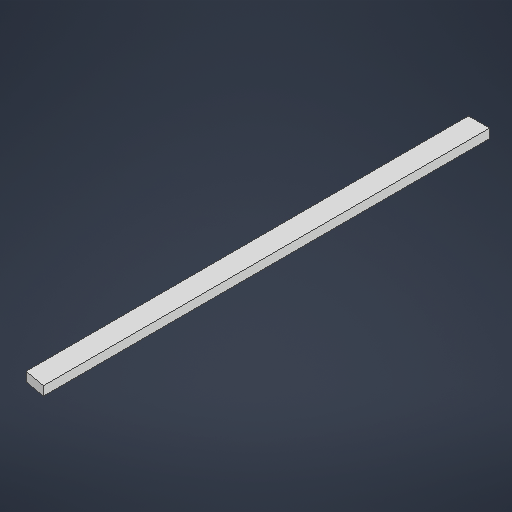
# Autodesk Inventor part: S_2x4x82
Saved by Autodesk Inventor 2027.1 (Build 311270010, 270A)
## iProperties
Created: 2026-09-01
Part Number: S_2x4x82
Material: Generic
Document SubType Name: Modeling
Designer: jorda
Density: 1 g/cm^3
Appearance: Default
Author: jorda
Autodesk Inventor part; units mm, degrees
ref_plane "YZ Plane" through (0, 0, 0) normal (1, 0, 0) x (0, 1, 0)
ref_plane "XZ Plane" through (0, 0, 0) normal (0, 1, 0) x (-1, 0, 0)
ref_plane "XY Plane" through (0, 0, 0) normal (0, 0, 1) x (1, 0, 0)
sketch "Sketch1" plane through (0, 0, 0) normal (0, 1, 0) x (-1, 0, 0)
  line L0 (0, 0) -> (88.9, -15.6755)
  line L1 (0, 0) -> (117.2884, 0) construction
  line L2 (88.9, -15.6755) -> (88.9, -1873.25)
  line L3 (0, 0) -> (0, -1873.25)
  line L4 (0, -1873.25) -> (0, 0)
  line L5 (0, 0) -> (0, -1873.25)
  line L6 (0, -1873.25) -> (88.9, -1873.25)
  constraints: 14 end point, 1 horizontal, 1 parallel, 1 perpendicular
extrude "Extrusion1" add sketch "Sketch1" along normal blind 38.1
body "Solid1"
